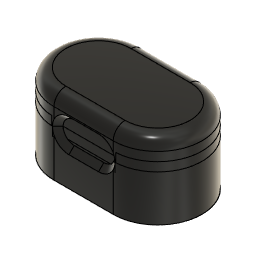
Sensoraufsatz (Autodesk Fusion 360 design; units mm, degrees)
Autodesk Fusion 360 part; units mm, degrees
sketch "Skizze1" plane through (0, 0, 0) normal (0, 0, 1) x (1, 0, 0)
  line L0 (0, 0) -> (20, 0)
  line L1 (20, 0) -> (20, 30)
  line L2 (20, 30) -> (0, 30)
  line L3 (0, 30) -> (0, 0)
  arc A0 (0, 30) -> (0, 0) centre (0, 15) ccw
  arc A1 (20, 0) -> (20, 30) centre (20, 15) ccw
  dimension "d1" = 20
  dimension "d2" = 30
  constraint coincident L0.start L3.end
  constraint horizontal L0
  constraint perpendicular L0 L1
  constraint perpendicular L1 L2
  constraint perpendicular L0 L3
  constraint tangent L0 A1
  measures "d1" distance of L0.start L0.end
  measures "d2" distance of L0.end L1.end
extrude "Extrusion1" add sketch "Skizze1" along normal blind 12.5 makes body 1
extrude "Extrusion2" add 1 faces at (13.3333, 10, 12.5) along direction (0, 0, 1) blind 10 separate body on bodies 1 makes body 2
shell "Schale1" thickness 3 removed faces 1 at (13.3333, 10, 12.5) on bodies 2
fillet "Abrundung1" radius 4 4 edges at (35, 15, 22.5) (10, 30, 22.5) (-15, 15, 22.5) (10, 0, 22.5) on bodies 2
sketch "Skizze2" plane through (0, 0, 0) normal (0, -1, 0) x (1, 0, 0)
  line L0 (20, 18.5) -> (0, 18.5)
  line L1 (0, 18.5) -> (0, 12.5)
  line L2 (0, 12.5) -> (20, 12.5)
  line L3 (20, 12.5) -> (20, 18.5)
  line L4 (7.5423, 16.2435) -> (5.0423, 16.2435)
  arc A0 (5.0423, 16.2435) -> (5.0423, 8.7435) centre (5.0423, 12.4935) ccw
  line L5 (5.0423, 8.7435) -> (15.0423, 8.7435)
  arc A1 (15.0423, 8.7435) -> (15.0423, 16.2435) centre (15.0423, 12.4935) ccw
  line L6 (15.0423, 16.2435) -> (7.5423, 16.2435)
  constraint horizontal L4
  constraint tangent L4 A0
  constraint tangent A0 L5
  constraint parallel L4 L5
  constraint tangent L5 A1
  constraint tangent A1 L6
extrude "Extrusion3" cut sketch "Skizze2" against normal blind 1.8 contours L2 L4 A0 A1 L6 bodies 2
sketch "Skizze3" plane through (0, 0, 0) normal (0, -1, 0) x (1, 0, 0)
  line L0 (0, 0) -> (20, 0)
  line L1 (20, 0) -> (20, 12.5)
  line L2 (20, 12.5) -> (0, 12.5)
  line L3 (0, 12.5) -> (0, 0)
  line L4 (5.0423, 16.2435) -> (15.0423, 16.2435)
  arc A0 (1.2927, 12.5) -> (5.0423, 8.757) centre (5.0423, 12.5066) ccw
  line L5 (5.0423, 8.757) -> (15.0423, 8.757)
  arc A1 (15.0423, 8.757) -> (18.7924, 12.5) centre (15.0423, 12.5071) ccw
  dimension "d17" = 3.7435
  constraint coincident L2 A0.start
  constraint tangent A0 L5
  constraint parallel L2 L5
  constraint coincident L2 A1.end
  constraint tangent L5 A1
  measures "d17" distance of L2 L4
extrude "Extrusion4" cut sketch "Skizze3" against normal blind 1.8 contours L2 A0 L5 A1 bodies 1
ref_plane "Arbeitsebene1" through (10, 15, 17.5) normal (0, -1, 0) x (1, 0, 0)
mirror "Spiegeln1" about plane through (10, 15, 17.5) normal (0, -1, 0) of "Extrusion3", "Extrusion4"
chamfer "Fase1" distance 1.8 angle 45 6 edges at (10.0423, 0, 16.2435) (2.393, 0, 15.1474) (17.6916, 0, 15.1474) (2.3932, 0, 9.8529) (17.6915, 0, 9.8529) (10.0423, 0, 8.757) on bodies 1 2
chamfer "Fase2" distance 1.8 angle 45 6 edges at (10.0423, 30, 16.2435) (17.6916, 30, 15.1474) (2.393, 30, 15.1474) (17.6915, 30, 9.8529) (2.3932, 30, 9.8529) (10.0423, 30, 8.757) on bodies 1 2
chamfer "Fase3" distance 4 angle 45 4 edges at (-12, 15, 19.5) (10, 3, 19.5) (32, 15, 19.5) (10, 27, 19.5) on bodies 2
sketch "Skizze4" plane through (0, 0, 12.5) normal (0, 0, 1) x (-1, 0, 0)
  line L0 (0.499, -29.9917) -> (-1.2927, -28.2)
  arc A0 (0.499, -29.9917) -> (0.499, -0.0083) centre (0, -15) ccw
  line L1 (-1.2927, -1.8) -> (0.499, -0.0083)
  line L2 (-1.2927, -1.8) -> (-18.7924, -1.8)
  line L3 (-20.5812, -0.0113) -> (-18.7924, -1.8)
  arc A1 (-20.5812, -0.0113) -> (-20.5812, -29.9887) centre (-20, -15) ccw
  line L4 (-18.7924, -28.2) -> (-20.5812, -29.9887)
  line L5 (-18.7924, -28.2) -> (-1.2927, -28.2)
  line L6 (-10, -12) -> (-18, -12)
  arc A2 (-18, -12) -> (-18, -18) centre (-18, -15) ccw
  line L7 (-18, -18) -> (-2.3671, -18)
  line L8 (-3, -12) -> (-10, -12)
  line L9 (-2.3671, -12) -> (-3, -12)
  arc A3 (-2.3671, -18) -> (-2.3671, -12) centre (-2.3671, -15) ccw
  dimension "d29" = 6
  dimension "d30" = 10.2
  dimension "d31" = 10.2
  constraint horizontal L6
  constraint tangent L6 A2
  constraint tangent A2 L7
  constraint parallel L6 L7
  constraint parallel L7 L9
  constraint tangent L9 A3
  constraint tangent L7 A3
  measures "d29" distance of L6 L7
  measures "d30" distance of L2 L6.start
  measures "d31" distance of L5 L7
extrude "Extrusion5" cut sketch "Skizze4" against normal blind 28 contours L6 A2 L7 L8 L9 A3 bodies 1
chamfer "Fase4" distance 2 angle 45 4 edges at (10.1835, 12, 12.5) (-0.6329, 15, 12.5) (10.1835, 18, 12.5) (21, 15, 12.5) on bodies 1
chamfer "Fase5" distance 2 angle 45 4 edges at (10.1835, 18, 0) (-0.6329, 15, 0) (10.1835, 12, 0) (21, 15, 0) on bodies 1
copy_body "Körper->Berechn1" bodies 1 removing the originals makes body 3 in component "Component"
copy_body "Körper->Berechn2" bodies 2 removing the originals makes body 4 in component "Component'"
sketch "Skizze8" plane through (0, 0, 12.5) normal (0, 0, -1) x (1, 0, 0)
  line L0 (20.581, -29.9887) -> (18.7923, -28.2)
  arc A0 (20.581, -29.9887) -> (20.581, -0.0113) centre (20, -15) ccw
  line L1 (18.7923, -1.8) -> (20.581, -0.0113)
  line L2 (18.7923, -1.8) -> (1.2923, -1.8)
  line L3 (-0.4994, -0.0083) -> (1.2923, -1.8)
  arc A1 (-0.4994, -0.0083) -> (-0.4994, -29.9917) centre (0, -15) ccw
  line L4 (1.2923, -28.2) -> (-0.4994, -29.9917)
  line L5 (1.2923, -28.2) -> (18.7923, -28.2)
  line L6 (0, -3) -> (20, -3)
  arc A2 (20, -27) -> (20, -3) centre (20, -15) ccw
  line L7 (20, -27) -> (0, -27)
  arc A3 (0, -3) -> (0, -27) centre (0, -15) ccw
sketch "Skizze9" plane through (0, 0, 12.5) normal (0, 0, 1) x (-1, 0, 0)
  line L0 (0.499, -29.9917) -> (-1.2927, -28.2)
  arc A0 (0.499, -29.9917) -> (0.499, -0.0083) centre (0, -15) ccw
  line L1 (-1.2927, -1.8) -> (0.499, -0.0083)
  line L2 (-1.2927, -1.8) -> (-18.7924, -1.8)
  line L3 (-20.5812, -0.0113) -> (-18.7924, -1.8)
  arc A1 (-20.5812, -0.0113) -> (-20.5812, -29.9887) centre (-20, -15) ccw
  line L4 (-18.7924, -28.2) -> (-20.5812, -29.9887)
  line L5 (-18.7924, -28.2) -> (-1.2927, -28.2)
  line L6 (-2.3671, -20) -> (-18, -20)
  arc A2 (-18, -10) -> (-18, -20) centre (-18, -15) ccw
  line L7 (-18, -10) -> (-2.3671, -10)
  line L8 (-3, -4) -> (-18, -4)
  line L9 (-18, -4) -> (-18, -4.4121)
  line L10 (-18, -8) -> (-3.0085, -8)
  line L11 (-3, -26) -> (-18, -26)
  line L12 (-17.3432, -22) -> (-2.9997, -22)
  arc A3 (-18, -4) -> (-18, -26) centre (-18, -15) ccw
  arc A4 (-3, -26) -> (-3, -4) centre (-3, -15) ccw
  line L13 (-18, -22) -> (-17.3432, -22)
  arc A5 (-18, -8) -> (-18, -22) centre (-18, -15) ccw
  arc A6 (-2.3671, -20) -> (-2.3671, -10) centre (-2.3671, -15) ccw
  line L14 (-3.0085, -8) -> (-2.3671, -8)
  line L15 (-2.3671, -22) -> (-2.9997, -22)
  arc A7 (-2.3671, -22) -> (-2.3671, -8) centre (-2.3671, -15) ccw
  dimension "d106" = 2
  dimension "d107" = 2
  constraint perpendicular L8 L9
  constraint tangent L8 A3
  constraint tangent L11 A3
  constraint tangent L11 A4
  constraint parallel L12 L13
  constraint tangent L10 A5
  constraint parallel L7 L14
  constraint parallel L12 L15
  constraint tangent L15 A7
  measures "d106" distance of L6 L12
  measures "d107" distance of L7 L10
extrude "Extrusion2'" cut sketch "Skizze9" against normal blind 4 contours L8 L11 A3 A4 bodies 3 in component "Component"
chamfer "Fase1'" distance 1 angle 45 4 edges at (-8, 15, 12.5) (10.5, 26, 12.5) (29, 15, 12.5) (10.5, 4, 12.5) on bodies 3 in component "Component"
sketch "Skizze10" plane through (0, 0, 12.5) normal (0, 0, 1) x (-1, 0, 0)
  line L0 (0.499, -29.9917) -> (-1.2927, -28.2)
  arc A0 (0.499, -29.9917) -> (0.499, -0.0083) centre (0, -15) ccw
  line L1 (-1.2927, -1.8) -> (0.499, -0.0083)
  line L2 (-1.2927, -1.8) -> (-18.7924, -1.8)
  line L3 (-20.5812, -0.0113) -> (-18.7924, -1.8)
  arc A1 (-20.5812, -0.0113) -> (-20.5812, -29.9887) centre (-20, -15) ccw
  line L4 (-18.7924, -28.2) -> (-20.5812, -29.9887)
  line L5 (-18.7924, -28.2) -> (-1.2927, -28.2)
  arc A2 (-3, -27) -> (-3, -3) centre (-3, -15) ccw
  line L6 (-3, -27) -> (-18, -27)
  arc A3 (-18, -3) -> (-18, -27) centre (-18, -15) ccw
  line L7 (-18, -3) -> (-3, -3)
  line L8 (-21.25, -2.0334) -> (-21.3322, -0.0593)
  line L9 (-21.25, -27.9666) -> (-20.8858, -27.9666)
  line L10 (-21.25, -27.9666) -> (-21.3307, -29.9409)
  line L11 (-20.5812, -29.9887) -> (-21.25, -27.9666)
  line L12 (0.499, -29.9917) -> (1.25, -27.9663)
  line L13 (1.25, -27.9663) -> (1.25, -29.9478)
  line L14 (1.25, -27.9663) -> (-10.5085, -27.9663)
  line L15 (1.25, -2.0264) -> (1.25, -0.0522)
  line L16 (-19.9999, -2.0334) -> (-1, -2.0264)
  line L17 (-10.5085, -27.9663) -> (-10.5222, -27.9666)
  line L18 (-20.8312, -29.977) -> (-21.25, -27.9666)
  line L19 (1.25, -27.9663) -> (0.7488, -29.9813)
  line L20 (1.25, -2.0264) -> (0.7488, -0.0187)
  line L21 (-21.25, -2.0334) -> (-20.8309, -0.023)
  line L22 (-20.8858, -27.9666) -> (-10.5222, -27.9666)
  line L23 (-21.25, -2.0334) -> (-19.9999, -2.0334)
  line L24 (-1, -2.0264) -> (1.25, -2.0264)
  line L25 (-20.5812, -0.0113) -> (-21.25, -2.0334)
  arc A4 (-21.25, -2.0334) -> (-21.25, -27.9666) centre (-21.25, -15) ccw
  arc A5 (1.25, -27.9663) -> (1.25, -2.0264) centre (1.25, -14.9963) ccw
  line L26 (1.25, -2.0264) -> (0.499, -0.0083)
  dimension "d94" = 22.5
  dimension "d96" = 0.751
  dimension "d97" = 0.751
  dimension "d98" = 0.25
  dimension "d99" = 0.25
  dimension "d100" = 0.751
  dimension "d101" = 0.25
  dimension "d102" = 0.751
  dimension "d103" = 0.25
  constraint coincident A1 L8.end
  constraint coincident A1 L10.end
  constraint coincident A1.end L4.end
  constraint coincident L0.start A0.start
  constraint coincident A0 L13.end
  constraint perpendicular L13 L14
  constraint coincident A0 L15.end
  constraint coincident A1 L18.start
  constraint coincident A0 L19.end
  constraint coincident A0 L20.end
  constraint coincident A1 L21.end
  constraint parallel L14 L22
  constraint horizontal L23
  constraint perpendicular L15 L24
  constraint coincident L3.start A1.start
  constraint tangent L23 A4
  constraint tangent L14 A5
  constraint coincident A0.end L1.end
  measures "d94" horizontal distance of L8.start L15.start
  measures "d96" distance of L10.end A1.end
  measures "d97" horizontal distance of L0.start L13.end
  measures "d98" horizontal distance of A1.end L18.start
  measures "d99" distance of L0.start L19.end
  measures "d100" horizontal distance of A0.end L15.end
  measures "d101" distance of A0.end L20.end
  measures "d102" horizontal distance of L8.end L3.start
  measures "d103" distance of L21.end L3.start
extrude "Extrusion9" [suppressed]
extrude "Extrusion3'" add sketch "Skizze10" along normal blind 3 contours A0 L13 L19 | A0 L13 L15 A5 | A0 L15 L20 | A1 L10 L18 | A1 L8 L10 A4 | A1 L8 L21 bodies 3 in component "Component"
sketch "Skizze11" plane through (0, 0, 12.5) normal (0, 0, -1) x (1, 0, 0)
  line L0 (20.581, -29.9887) -> (18.7923, -28.2)
  arc A0 (20.581, -29.9887) -> (20.581, -0.0113) centre (20, -15) ccw
  line L1 (18.7923, -1.8) -> (20.581, -0.0113)
  line L2 (18.7923, -1.8) -> (1.2923, -1.8)
  line L3 (-0.4994, -0.0083) -> (1.2923, -1.8)
  arc A1 (-0.4994, -0.0083) -> (-0.4994, -29.9917) centre (0, -15) ccw
  line L4 (1.2923, -28.2) -> (-0.4994, -29.9917)
  line L5 (1.2923, -28.2) -> (18.7923, -28.2)
  line L6 (0, -3) -> (20, -3)
  arc A2 (20, -27) -> (20, -3) centre (20, -15) ccw
  line L7 (20, -27) -> (0, -27)
  arc A3 (0, -3) -> (0, -27) centre (0, -15) ccw
  line L8 (20.581, -0.0113) -> (21, -2.5)
  line L9 (-0.4994, -0.0083) -> (-1, -2.5)
  line L10 (-1, -2.5) -> (21, -2.5)
  line L11 (-0.4994, -29.9917) -> (-1, -27.5)
  line L12 (-1, -27.5) -> (21, -27.5)
  line L13 (21, -27.5) -> (20.581, -29.9887)
  arc A4 (21, -27.5) -> (21, -2.5) centre (21, -15) ccw
  arc A5 (-1, -2.5) -> (-1, -27.5) centre (-1, -15) ccw
  constraint coincident A0.end L1.end
  constraint coincident L3.start A1.start
  constraint horizontal L10
  constraint coincident A1.end L4.end
  constraint horizontal L12
  constraint coincident L0.start A0.start
  constraint tangent L12 A4
  constraint tangent L10 A4
  constraint tangent L10 A5
  constraint tangent L12 A5
extrude "Extrusion10" [suppressed]
extrude "Extrusion1'" add sketch "Skizze11" along normal blind 3 contours L0 L4 L5 L11 L12 L13 | L1 L2 L3 L8 L9 L10 | L10 L12 A4 A5 bodies 4 in component "Component'"
sketch "Skizze12" plane through (0, 0, 12.5) normal (0, 0, 1) x (-1, 0, 0)
  line L0 (0.499, -29.9917) -> (-1.2927, -28.2)
  arc A0 (0.499, -29.9917) -> (0.7488, -29.9813) centre (0, -15) ccw
  line L1 (-1.2927, -1.8) -> (0.499, -0.0083)
  line L2 (-1.2927, -1.8) -> (-18.7924, -1.8)
  line L3 (-20.5812, -0.0113) -> (-18.7924, -1.8)
  arc A1 (-20.8312, -29.977) -> (-20.5812, -29.9887) centre (-20, -15) ccw
  line L4 (-18.7924, -28.2) -> (-20.5812, -29.9887)
  line L5 (-18.7924, -28.2) -> (-1.2927, -28.2)
  arc A2 (-3, -27) -> (-3, -3) centre (-3, -15) ccw
  line L6 (-3, -27) -> (-18, -27)
  arc A3 (-18, -3) -> (-18, -27) centre (-18, -15) ccw
  line L7 (-18, -3) -> (-3, -3)
  line L8 (-21.25, -27.9666) -> (-20.8312, -29.977)
  line L9 (0.7488, -29.9813) -> (1.25, -27.9663)
  arc A4 (1.25, -27.9663) -> (1.25, -2.0264) centre (1.25, -14.9963) ccw
  line L10 (1.25, -2.0264) -> (0.7488, -0.0187)
  arc A5 (0.7488, -0.0187) -> (0.499, -0.0083) centre (0, -15) ccw
  arc A6 (-20.5812, -0.0113) -> (-20.8309, -0.023) centre (-20, -15) ccw
  line L11 (-20.8309, -0.023) -> (-21.25, -2.0334)
  arc A7 (-21.25, -2.0334) -> (-21.25, -27.9666) centre (-21.25, -15) ccw
sketch "Skizze13" plane through (0, 0, 0) normal (0, 0, -1) x (1, 0, 0)
  arc A0 (20, -30) -> (20, 0) centre (20, -15) ccw
  line L0 (20, 0) -> (0, 0)
  arc A1 (0, 0) -> (0, -30) centre (0, -15) ccw
  line L1 (0, -30) -> (20, -30)
  line L2 (2.3671, -10) -> (18, -10)
  arc A2 (18, -20) -> (18, -10) centre (18, -15) ccw
  line L3 (18, -20) -> (2.3671, -20)
  line L4 (0, -1.5) -> (20.0344, -1.5)
  arc A3 (20, -28.4005) -> (20.0344, -1.5) centre (20.0344, -14.9503) ccw
  line L5 (20, -28.4005) -> (0, -28.4005)
  arc A4 (0, -1.5) -> (0, -28.4005) centre (0, -14.9502) ccw
  arc A5 (2.3671, -10) -> (2.3671, -20) centre (2.3671, -15) ccw
  constraint parallel L0 L4
  constraint tangent L4 A3
  constraint parallel L4 L5
  constraint tangent L5 A4
  constraint tangent L4 A4
extrude "Extrusion11" [suppressed]
extrude "Extrusion4'" add sketch "Skizze13" along normal blind 3 contours A0 L0 A1 L1 bodies 3 in component "Component"
chamfer "Fase2'" distance 2 angle 45 4 edges at (-4.6329, 15, 12.5) (10.1835, 8, 12.5) (25, 15, 12.5) (10.1835, 22, 12.5) on bodies 3 in component "Component"
fillet "Abrundung2" radius 1.5 4 edges at (10, 28.4005, -3) (-13.4502, 14.9502, -3) (10.0172, 1.5, -3) (33.4847, 14.9675, -3) on bodies 3 in component "Component"
component "Component" placed x (1, 0, 0) y (0, 1, 0) z (0, 0, 1) at (0, 0, 0)
component "Component'" placed x (1, 0, 0) y (0, 1, 0) z (0, 0, 1) at (0, 0, 0)
